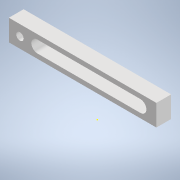
# Autodesk Inventor part: cover-holder2
Saved by Autodesk Inventor 2020 (Build 240168000, 168)
## iProperties
Created: 2019-11-14
Part Number: cover-holder2
Material: Generic
Document SubType Name: Modeling
Designer: Hymowitz
Density: 1 g/cm^3
Appearance: Default
Author: Hymowitz
Autodesk Inventor part; units mm, degrees
ref_plane "YZ Plane" through (0, 0, 0) normal (1, 0, 0) x (0, 1, 0)
ref_plane "XZ Plane" through (0, 0, 0) normal (0, 1, 0) x (-1, 0, 0)
ref_plane "XY Plane" through (0, 0, 0) normal (0, 0, 1) x (1, 0, 0)
sketch "Sketch1" plane through (0, 0, 0) normal (0, 0, 1) x (1, 0, 0)
  line L0 (-22.235, -36.3697) -> (-22.235, -26.7755) projected
  line L1 (-22.235, -26.7755) -> (-25.9663, -26.7755) projected
  line L2 (-26.045, -26.8374) -> (-26.045, -30.1399) projected
  arc A0 (-26.045, -30.1399) -> (-26.045, -34.0927) centre (-24.7167, -32.1163) ccw projected
  line L3 (-26.045, -34.0927) -> (-26.045, -36.3697) projected
  line L4 (-26.045, -36.3697) -> (-31.75, -36.3697) projected
  line L5 (-31.75, -36.3697) -> (-31.75, -19.7975) projected
  line L6 (-31.75, -19.7975) -> (31.75, -19.7975) projected
  line L7 (31.75, -19.7975) -> (31.75, -36.3697) projected
  line L8 (31.75, -36.3697) -> (-22.235, -36.3697) projected
  line L9 (24.7167, -22.9725) -> (-19.6375, -22.9725) projected
  arc A1 (-19.6375, -22.9725) -> (-19.6375, -28.1475) centre (-19.6375, -25.56) ccw projected
  line L10 (-19.6375, -28.1475) -> (24.7167, -28.1475) projected
  arc A2 (24.7167, -28.1475) -> (24.7167, -22.9725) centre (24.7167, -25.56) ccw projected
  line L11 (-18.6822, -29.735) -> (-18.6822, -34.4975) projected
  line L12 (-18.6822, -34.4975) -> (24.7167, -34.4975) projected
  arc A3 (24.7167, -34.4975) -> (24.7167, -29.735) centre (24.7167, -32.1163) ccw projected
  line L13 (24.7167, -29.735) -> (-18.6822, -29.735) projected
  line L14 (-31.75, 25.8027) -> (31.75, 25.8027)
  line L15 (31.75, 25.8027) -> (31.75, 15.6277)
  line L16 (31.75, 15.6277) -> (-31.75, 15.6277)
  line L17 (-31.75, 15.6277) -> (-31.75, 25.8027)
  circle A4 centre (-26.9875, 20.7152) radius 1.5875
  line L18 (-26.9875, 20.7152) -> (-26.9875, 4.175)
  line L19 (-19.4952, 20.7152) -> (24.859, 20.7152) construction
  line L20 (-19.4952, 18.1277) -> (24.859, 18.1277)
  line L21 (24.859, 23.3027) -> (-19.4952, 23.3027)
  arc A5 (-19.4952, 23.3027) -> (-19.4952, 18.1277) centre (-19.4952, 20.7152) ccw
  arc A6 (24.859, 18.1277) -> (24.859, 23.3027) centre (24.859, 20.7152) ccw
  line L22 (12.1015, 23.3027) -> (12.1015, 18.1277) construction
  line L23 (12.1015, -22.9725) -> (12.1015, -28.1475) construction
  line L24 (-31.75, 20.7152) -> (-23.8125, 20.7152) construction
  arc A7 (-25.9663, -26.7755) -> (-26.045, -26.8374) centre (-26.9875, -25.56) ccw projected
  point P0 (0, 0)
  point P1 (2.6819, 20.7152)
  dimension "d0" = 2.5
  dimension "d5" = 44.3542
  constraints: 24 end point, 5 point on line, 4 collinear, 4 point on circle, 4 tangent, 3 centre point, 3 horizontal, 3 parallel, 3 perpendicular, 2 midpoint, 1 equal radius, 1 vertical
  measures "d0" distance between parallel lines of L16 L20
  measures "d5" distance of L19.start L19.end
ref_plane "Work Plane1" through (-31.75, -10.525, -6.35) normal (0, 0, -1) x (0, 1, 0)
extrude "Extrusion1" add sketch "Sketch1" against normal up to surface (6.35 mm away) contours L14 L15 L16 L17
sketch "Sketch2" plane through (31.75, 15.6277, -6.35) normal (0, 0, -1) x (-1, 0, 0)
  point P0 (31.75, -15.6277)
sketch "Sketch3" plane through (-31.75, 25.8027, 0) normal (0, 1, 0) x (1, 0, 0)
  line L0 (0.254, -20.066) -> (0.254, 30.48) projected
  arc A0 (6.604, 36.83) -> (0.254, 30.48) centre (6.604, 30.48) ccw projected
  line L1 (6.604, 36.83) -> (57.15, 36.83) projected
  arc A1 (63.5, 30.48) -> (57.15, 36.83) centre (57.15, 30.48) ccw projected
  line L2 (63.5, -20.066) -> (63.5, 30.48) projected
  arc A2 (57.15, -26.416) -> (63.5, -20.066) centre (57.15, -20.066) ccw projected
  line L3 (6.604, -26.416) -> (57.15, -26.416) projected
  arc A3 (0.254, -20.066) -> (6.604, -26.416) centre (6.604, -20.066) ccw projected
  circle A4 centre (59.817, 30.607) radius 1.4732 projected
  circle A5 centre (3.937, 30.607) radius 1.4732 projected
  circle A6 centre (59.817, -20.193) radius 1.4732 projected
  circle A7 centre (3.937, -20.193) radius 1.4732 projected
  line L4 (63.5, 0) -> (0, 0) projected
  line L5 (0, 0) -> (63.5, 0) projected
  line L6 (9.0714, 0) -> (22.6786, 0)
  line L7 (22.6786, 0) -> (22.6786, -7.9375)
  line L8 (22.6786, -7.9375) -> (9.0714, -7.9375)
  line L9 (9.0714, -7.9375) -> (9.0714, 0)
  line L10 (63.5, 6.35) -> (0, 6.35) projected
  line L11 (22.6786, 6.35) -> (9.0714, 6.35)
  line L12 (9.0714, 6.35) -> (9.0714, 12.7)
  line L13 (9.0714, 12.7) -> (22.6786, 12.7)
  line L14 (22.6786, 12.7) -> (22.6786, 6.35)
  line L15 (56.2674, 0) -> (42.6602, 0)
  line L16 (42.6602, 0) -> (42.6602, -7.9375)
  line L17 (42.6602, -7.9375) -> (56.2674, -7.9375)
  line L18 (56.2674, -7.9375) -> (56.2674, 0)
  line L19 (0, 6.35) -> (63.5, 6.35) projected
  line L20 (56.2674, 6.35) -> (42.6602, 6.35)
  line L21 (42.6602, 6.35) -> (42.6602, 14.2875)
  line L22 (42.6602, 14.2875) -> (56.2674, 14.2875)
  line L23 (56.2674, 14.2875) -> (56.2674, 6.35)
  point P0 (31.75, 0)
  constraints: 32 end point, 9 point on line, 8 parallel, 4 horizontal, 4 perpendicular, 2 collinear
extrude "Extrusion2" add sketch "Sketch3" against normal blind 1.5875 contours L4 L7 L8 L9 | L12 L13 L14 L10 | L4 L18 L17 L16 | L21 L22 L23 L10
body "Solid1"
